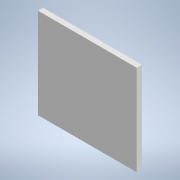
# Autodesk Inventor part: Palma
Saved by Autodesk Inventor 2020.4 (Build 244396010, 396A)
## iProperties
Created: 2021-09-01
Part Number: Palma
Material: Generic
Document SubType Name: Modeling
Designer: chalo
Density: 1 g/cm^3
Appearance: Default
Author: chalo
Autodesk Inventor part; units mm, degrees
ref_plane "YZ Plane" through (0, 0, 0) normal (1, 0, 0) x (0, 1, 0)
ref_plane "XZ Plane" through (0, 0, 0) normal (0, 1, 0) x (-1, 0, 0)
ref_plane "XY Plane" through (0, 0, 0) normal (0, 0, 1) x (1, 0, 0)
sketch "Sketch1" plane through (0, 0, 0) normal (0, 0, 1) x (1, 0, 0)
  line L0 (-4.4, 49.4) -> (30, 49.4) projected
  line L1 (-4.4, -37.6) -> (30, -37.6) projected
  line L2 (-4.4, -37.6) -> (90.6, -37.6)
  line L3 (90.6, -37.6) -> (90.6, 49.4)
  line L4 (90.6, 49.4) -> (-4.4, 49.4)
  line L5 (-4.4, 49.4) -> (-4.4, -37.6)
  point P0 (0, 0)
  dimension "d0" = 95
  constraints: 8 end point, 2 parallel, 1 horizontal, 1 perpendicular
  measures "d0" distance of L0.start L3.end
extrude "Extrusion1" add sketch "Sketch1" against normal blind 3
body "Solid1"
